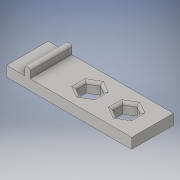
# Autodesk Inventor part: Gap Guage
Saved by Autodesk Inventor 2016 (Build 200138000, 138)
## iProperties
Created: 2015-07-12
Part Number: Gap Guage
Material: Generic
Document SubType Name: Modeling
Designer: steele
Density: 1 g/cm^3
Appearance: Default
Author: steele
Autodesk Inventor part; units mm, degrees
ref_plane "YZ Plane" through (0, 0, 0) normal (1, 0, 0) x (0, 1, 0)
ref_plane "XZ Plane" through (0, 0, 0) normal (0, 1, 0) x (-1, 0, 0)
ref_plane "XY Plane" through (0, 0, 0) normal (0, 0, 1) x (1, 0, 0)
sketch "Sketch1" plane through (0, 0, 0) normal (0, 1, 0) x (-1, 0, 0)
  line L0 (-76.2, 25.4) -> (-76.2, -25.4)
  line L1 (-76.2, -25.4) -> (76.2, -25.4)
  line L2 (76.2, -25.4) -> (76.2, 25.4)
  line L3 (76.2, 25.4) -> (-76.2, 25.4)
  line L4 (-76.2, 25.4) -> (76.2, -25.4) construction
  line L5 (-76.2, -25.4) -> (76.2, 25.4) construction
  point P0 (0, 0)
  dimension "d0" = 50.8
  dimension "d1" = 152.4
  constraints: 12 end point, 2 midpoint, 2 parallel, 1 perpendicular, 1 vertical
  measures "d0" distance of L0.start L0.end
  measures "d1" distance of L2.end L0.start
extrude "Extrusion1" add sketch "Sketch1" against normal blind 12.7
sketch "Sketch2" plane through (0, 0, 0) normal (0, 1, 0) x (1, 0, 0)
  line L0 (-47.625, -25.4) -> (-47.625, 25.4)
  line L1 (-47.625, 25.4) -> (-53.975, 25.4)
  line L2 (-53.975, 25.4) -> (-53.975, -25.4)
  line L3 (-53.975, -25.4) -> (-47.625, -25.4)
  line L4 (-47.625, -25.4) -> (-53.975, 25.4) construction
  line L5 (-47.625, 25.4) -> (-53.975, -25.4) construction
  line L6 (-76.2, 25.4) -> (-76.2, -25.4) projected
  point P0 (0, 0)
  point P1 (-50.8, 0)
  dimension "d4" = 6.35
  dimension "d5" = 25.4
  dimension "d6" = 50.8
  constraints: 12 end point, 2 midpoint, 2 parallel, 1 perpendicular, 1 vertical
  measures "d4" distance between parallel lines of L2 L0
  measures "d5" distance from line of L6 point (-50.8, 0)
  measures "d6" distance of L1.end L2.end
extrude "Extrusion2" add sketch "Sketch2" along normal blind 11.1125
fillet "Fillet1" radius 3.175 2 edges at (-47.625, 11.1125, 0) (-53.975, 11.1125, 0)
sketch "Sketch3" plane through (0, 0, 0) normal (0, 1, 0) x (1, 0, 0)
  line L0 (33.4515, -6.1606) -> (33.4515, 6.5394)
  line L1 (33.4515, 6.5394) -> (44.45, 12.8894)
  line L2 (44.45, 12.8894) -> (55.4485, 6.5394)
  line L3 (55.4485, 6.5394) -> (55.4485, -6.1606)
  line L4 (55.4485, -6.1606) -> (44.45, -12.5106)
  line L5 (44.45, -12.5106) -> (33.4515, -6.1606)
  line L6 (-10.9985, -6.35) -> (-10.9985, 6.35)
  line L7 (-10.9985, 6.35) -> (0, 12.7)
  line L8 (0, 12.7) -> (10.9985, 6.35)
  line L9 (10.9985, 6.35) -> (10.9985, -6.35)
  line L10 (10.9985, -6.35) -> (0, -12.7)
  line L11 (0, -12.7) -> (-10.9985, -6.35)
  line L12 (73.025, 22.225) -> (73.025, -22.225) projected
  point P0 (0, 0)
  point P1 (44.45, 0.1894)
  point P2 (0, 0)
  dimension "d12" = 25.4
  dimension "d13" = 44.45
  constraints: 24 end point, 3 parallel, 1 coincident, 26 other
  measures "d12" distance of L1.end L4.end
  measures "d13" horizontal distance of point (44.45, 0.189) point (0, 0)
extrude "Extrusion3" cut sketch "Sketch3" against normal through all
fillet "Fillet4" radius 3.175 12 edges at (49.9493, 0, 9.3356) (38.9507, 0, 9.3356) (33.4515, 0, -0.1894) (38.9507, 0, -9.7144) (49.9493, 0, -9.7144) (55.4485, 0, -0.1894) (10.9985, 0, 0) (5.4993, 0, 9.525) (-5.4993, 0, 9.525) (-10.9985, 0, 0) (-5.4993, 0, -9.525) (5.4993, 0, -9.525)
body "Solid1"
